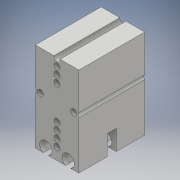
# Autodesk Inventor part: wirst fix
Saved by Autodesk Inventor 2017 (Build 210142000, 142)
## iProperties
Created: 2016-12-10
Part Number: wirst fix
Material: Generic
Document SubType Name: Modeling
Designer: Bardo91
Density: 1 g/cm^3
Appearance: Default
Author: Bardo91
Autodesk Inventor part; units mm, degrees
ref_plane "YZ Plane" through (0, 0, 0) normal (1, 0, 0) x (0, 1, 0)
ref_plane "XZ Plane" through (0, 0, 0) normal (0, 1, 0) x (-1, 0, 0)
ref_plane "XY Plane" through (0, 0, 0) normal (0, 0, 1) x (1, 0, 0)
sketch "Sketch1" plane through (0, 0, 0) normal (0, 0, 1) x (1, 0, 0)
  line L0 (0, 0) -> (19.5, 0)
  line L1 (19.5, 0) -> (19.5, 29.5)
  line L2 (19.5, 29.5) -> (0, 29.5)
  line L3 (0, 29.5) -> (0, 0)
  dimension "d0" = 19.5
  dimension "d1" = 29.5
  constraints: 8 end point, 2 horizontal, 2 perpendicular
  measures "d0" distance of L0.start L0.end
  measures "d1" distance of L0.end L1.end
extrude "Extrusion1" add sketch "Sketch1" along normal blind 40
sketch "Sketch2" plane through (0, 0, 0) normal (0, -1, 0) x (1, 0, 0)
  line L0 (0, 0) -> (19.5, 0) projected
  line L1 (9.75, 0) -> (9.75, 2.5)
  line L2 (9.75, 2.5) -> (14.75, 2.5)
  line L3 (14.75, 2.5) -> (4.75, 2.5)
  circle A0 centre (4.75, 2.5) radius 2.75
  circle A1 centre (14.75, 2.5) radius 2.75
  dimension "d4" = 2.5
  dimension "d5" = 5
  dimension "d6" = 10
  dimension "d7" = 5.5
  dimension "d8" = 5.5
  constraints: 6 end point, 2 centre point, 2 coincident, 1 midpoint, 1 perpendicular, 1 point on line, 1 vertical
  measures "d4" distance of L1.start L1.end
  measures "d5" distance of L1.end L2.end
  measures "d6" distance of L2.end L3.end
  measures "d7" diameter of A0
  measures "d8" diameter of A1
extrude "Extrusion2" cut sketch "Sketch2" against normal through all contours A0 L0 | L0 A0 | A1 L0 | L0 A1
sketch "Sketch3" plane through (0, 0, 0) normal (0, 0, -1) x (-1, 0, 0)
  line L0 (0, 29.5) -> (0, 0) projected
  line L1 (0, 14.75) -> (-19.5, 14.75)
  line L2 (-19.5, 0) -> (-19.5, 29.5) projected
  line L3 (-19.5, 14.75) -> (-19.5, 12.75)
  line L4 (-19.5, 12.75) -> (-19.5, 16.75)
  line L5 (-19.5, 16.75) -> (0, 16.75)
  line L6 (0, 16.75) -> (0, 12.75)
  line L7 (0, 12.75) -> (-19.5, 12.75)
  dimension "d11" = 2
  dimension "d12" = 4
  constraints: 12 end point, 2 midpoint, 2 perpendicular, 2 point on line, 1 parallel
  measures "d11" distance of L1.end L3.end
  measures "d12" distance of L3.end L4.end
extrude "Extrusion3" cut sketch "Sketch3" against normal blind 9
sketch "Sketch4" plane through (0, 0, 40) normal (0, -1, 0) x (1, 0, 0)
  line L0 (19.5, 0) -> (0, 0) projected
  line L1 (9.75, 0) -> (9.75, -17.5)
  line L2 (9.75, -17.5) -> (9.75, -10)
  circle A0 centre (9.75, -10) radius 1.375
  circle A1 centre (9.75, -6.75) radius 1.375
  circle A2 centre (9.75, -3.5) radius 1.375
  circle A3 centre (9.75, -0.25) radius 1.375
  circle A4 centre (2.25, -17.5) radius 1.375
  circle A5 centre (-1, -17.5) radius 1.375
  circle A6 centre (-4.25, -17.5) radius 1.375
  circle A7 centre (-7.5, -17.5) radius 1.375
  circle A8 centre (9.75, -25) radius 1.375
  circle A9 centre (9.75, -28.25) radius 1.375
  circle A10 centre (9.75, -31.5) radius 1.375
  circle A11 centre (9.75, -34.75) radius 1.375
  circle A12 centre (17.25, -17.5) radius 1.375
  circle A13 centre (20.5, -17.5) radius 1.375
  circle A14 centre (23.75, -17.5) radius 1.375
  circle A15 centre (27, -17.5) radius 1.375
  point P0 (0, -40)
  dimension "d15" = 17.5
  dimension "d16" = 7.5
  dimension "d17" = 2.75
  dimension "d20" = 3.25
  dimension "d27" = 360
  constraints: 16 centre point, 4 end point, 2 vertical, 1 coincident, 1 midpoint, 1 point on line, 39 other
  measures "d15" distance of L1.start L1.end
  measures "d16" distance of L1.end L2.end
  measures "d17" diameter of A0
  measures "d20" distance of A0.centre A1.centre
extrude "Extrusion4" cut sketch "Sketch4" against normal through all
body "Solid1"
